Autodesk Fusion 360 part; units mm, degrees
(part 39 of 40)
  line L11251 (159.0031, 181.5729) -> (158.8856, 181.6744) construction
  line L11252 (158.8856, 181.6744) -> (158.7686, 181.7767) construction
  line L11253 (158.7686, 181.7767) -> (158.6523, 181.88) construction
  line L11254 (158.6523, 181.88) -> (158.5369, 181.9844) construction
  line L11255 (158.5369, 181.9844) -> (158.4226, 182.0903) construction
  line L11256 (158.4226, 182.0903) -> (158.3096, 182.1981) construction
  line L11257 (158.3096, 182.1981) -> (158.198, 182.3077) construction
  line L11258 (158.198, 182.3077) -> (158.0876, 182.419) construction
  line L11259 (158.0876, 182.419) -> (157.9783, 182.5316) construction
  line L11260 (157.9783, 182.5316) -> (157.8698, 182.6455) construction
  line L11261 (157.8698, 182.6455) -> (157.7622, 182.7603) construction
  line L11262 (157.7622, 182.7603) -> (157.6553, 182.876) construction
  line L11263 (157.6553, 182.876) -> (157.5492, 182.9927) construction
  line L11264 (157.5492, 182.9927) -> (157.4439, 183.1105) construction
  line L11265 (157.4439, 183.1105) -> (157.3394, 183.2292) construction
  line L11266 (157.3394, 183.2292) -> (157.2359, 183.3491) construction
  line L11267 (157.2359, 183.3491) -> (157.1332, 183.47) construction
  line L11268 (157.1332, 183.47) -> (157.0313, 183.5919) construction
  line L11269 (157.0313, 183.5919) -> (156.9303, 183.7148) construction
  line L11270 (156.9303, 183.7148) -> (156.83, 183.8386) construction
  line L11271 (156.83, 183.8386) -> (156.7305, 183.9633) construction
  line L11272 (156.7305, 183.9633) -> (156.6317, 184.0888) construction
  line L11273 (156.6317, 184.0888) -> (156.5336, 184.2151) construction
  line L11274 (156.5336, 184.2151) -> (156.4363, 184.3423) construction
  line L11275 (156.4363, 184.3423) -> (156.3397, 184.4703) construction
  line L11276 (156.3397, 184.4703) -> (156.2439, 184.5991) construction
  line L11277 (156.2439, 184.5991) -> (156.1488, 184.7288) construction
  line L11278 (156.1488, 184.7288) -> (156.0544, 184.8592) construction
  line L11279 (156.0544, 184.8592) -> (155.9608, 184.9905) construction
  line L11280 (155.9608, 184.9905) -> (155.8678, 185.1224) construction
  line L11281 (155.8678, 185.1224) -> (155.7756, 185.2552) construction
  line L11282 (155.7756, 185.2552) -> (155.684, 185.3886) construction
  line L11283 (155.684, 185.3886) -> (155.5932, 185.5228) construction
  line L11284 (155.5932, 185.5228) -> (155.503, 185.6577) construction
  line L11285 (155.503, 185.6577) -> (155.4135, 185.7933) construction
  line L11286 (155.4135, 185.7933) -> (155.3247, 185.9295) construction
  line L11287 (155.3247, 185.9295) -> (155.2365, 186.0665) construction
  line L11288 (155.2365, 186.0665) -> (155.1491, 186.2042) construction
  line L11289 (155.1491, 186.2042) -> (155.0623, 186.3425) construction
  line L11290 (155.0623, 186.3425) -> (154.9762, 186.4815) construction
  line L11291 (154.9762, 186.4815) -> (154.8907, 186.6211) construction
  line L11292 (154.8907, 186.6211) -> (154.8059, 186.7614) construction
  line L11293 (154.8059, 186.7614) -> (154.7218, 186.9023) construction
  line L11294 (154.7218, 186.9023) -> (154.6383, 187.0438) construction
  line L11295 (154.6383, 187.0438) -> (154.5555, 187.186) construction
  line L11296 (154.5555, 187.186) -> (154.4733, 187.3288) construction
  line L11297 (154.4733, 187.3288) -> (154.3917, 187.4721) construction
  line L11298 (154.3917, 187.4721) -> (154.3108, 187.6161) construction
  line L11299 (154.3108, 187.6161) -> (154.2306, 187.7607) construction
  line L11300 (154.2306, 187.7607) -> (154.151, 187.9058) construction
  line L11301 (154.151, 187.9058) -> (154.072, 188.0515) construction
  line L11302 (154.072, 188.0515) -> (153.9937, 188.1978) construction
  line L11303 (153.9937, 188.1978) -> (153.916, 188.3447) construction
  line L11304 (153.916, 188.3447) -> (153.8389, 188.4921) construction
  line L11305 (153.8389, 188.4921) -> (153.7625, 188.6401) construction
  line L11306 (153.7625, 188.6401) -> (153.6867, 188.7886) construction
  line L11307 (153.6867, 188.7886) -> (153.6115, 188.9377) construction
  line L11308 (153.6115, 188.9377) -> (153.537, 189.0873) construction
  line L11309 (153.537, 189.0873) -> (153.463, 189.2374) construction
  line L11310 (153.463, 189.2374) -> (153.3897, 189.3881) construction
  line L11311 (153.3897, 189.3881) -> (153.3171, 189.5393) construction
  line L11312 (153.3171, 189.5393) -> (153.245, 189.6909) construction
  line L11313 (153.245, 189.6909) -> (153.1736, 189.8431) construction
  line L11314 (153.1736, 189.8431) -> (153.1169, 189.9653) construction
  line L11315 (153.1169, 189.9653) -> (153.0747, 190.0572) construction
  line L11316 (153.0747, 190.0572) -> (153.0467, 190.1185) construction
  line L11317 (153.0467, 190.1185) -> (153.0327, 190.1492) construction
  line L11318 (256.7226, 110.7517) -> (257.9473, 109.6737)
  line L11319 (154.1697, 136.995) -> (152.5778, 136.6378)
  line L11320 (154.1697, 163.005) -> (152.5778, 163.3622)
  line L11321 (217.6748, 90.8558) -> (217.8271, 89.2315)
  line L11322 (152.9878, 144.4572) -> (151.3635, 144.3049)
  line L11323 (225.137, 92.0377) -> (225.4942, 90.4458)
  line L11324 (266.6686, 173.5481) -> (268.1665, 174.1948)
  line L11325 (263.2386, 119.7202) -> (264.6423, 118.8885)
  line L11326 (270.0943, 136.995) -> (271.6862, 136.6378)
  line L11327 (242.4118, 201.1066) -> (243.2435, 202.5103)
  line L11328 (161.0254, 180.2798) -> (159.6217, 181.1115)
  line L11329 (154.1697, 136.995) -> (152.5778, 136.6378)
  arc A302 (172.7536, 191.8132) -> (172.8837, 194.5906) centre (171.3824, 193.2692) ccw
  arc A303 (199.127, 207.9623) -> (201.4504, 206.435) centre (201.0785, 208.4001) ccw
  arc A304 (204.8514, 206.9737) -> (206.5892, 209.1442) centre (204.5979, 208.9575) ccw
  arc A305 (239.7302, 200.3721) -> (242.4118, 201.1066) centre (240.6912, 202.1261) ccw
  arc A306 (266.6686, 126.4519) -> (264.0674, 125.4699) centre (265.8758, 124.6158) ccw
  arc A307 (256.7226, 110.7517) -> (253.9452, 110.6216) centre (255.4012, 109.2504) ccw
  spline S151 degree 5 poles (198.7698, 90.4458) (198.763, 90.4157) (198.7487, 90.3556) (198.7249, 90.2662) (198.6885, 90.1483) (198.6369, 90.0027) (198.5809, 89.8584) (198.5221, 89.7148) (198.4619, 89.5717) (198.4007, 89.4289) (198.3385, 89.2864) (198.2749, 89.1443) (198.2094, 89.0029) (198.1418, 88.8621) (198.072, 88.7221) (198.0004, 88.5827) (197.927, 88.4439) (197.8523, 88.3056) (197.7763, 88.1678) (197.6993, 88.0303) (197.6211, 87.8933) (197.5416, 87.7568) (197.4609, 87.6208) (197.379, 87.4852) (197.2957, 87.3502) (197.2112, 87.2157) (197.1256, 87.0816) (197.0388, 86.948) (196.951, 86.8148) (196.8622, 86.682) (196.7723, 86.5497) (196.6814, 86.4179) (196.5895, 86.2865) (196.4966, 86.1555) (196.4027, 86.025) (196.3078, 85.895) (196.212, 85.7654) (196.1152, 85.6362) (196.0174, 85.5074) (195.9188, 85.3791) (195.8193, 85.2512) (195.7189, 85.1238) (195.6176, 84.9968) (195.5154, 84.8702) (195.4124, 84.744) (195.3085, 84.6183) (195.2037, 84.493) (195.0982, 84.3682) (194.9918, 84.2438) (194.8846, 84.1198) (194.7765, 83.9962) (194.6677, 83.8731) (194.5581, 83.7503) (194.4478, 83.6281) (194.3366, 83.5062) (194.2247, 83.3848) (194.112, 83.2638) (193.9985, 83.1432) (193.8843, 83.0231) (193.7694, 82.9034) (193.6538, 82.7841) (193.5374, 82.6653) (193.4202, 82.5469) (193.3024, 82.4289) (193.1839, 82.3113) (193.0646, 82.1942) (192.9447, 82.0775) (192.8241, 81.9612) (192.7027, 81.8454) (192.5808, 81.73) (192.4581, 81.615) (192.3594, 81.5233) (192.2851, 81.4548) (192.2354, 81.4092) (192.2105, 81.3864) knots 0 0 0 0 0 0 0.01428571 0.02857143 0.04285714 0.05714286 0.07142857 0.08571429 0.1 0.11428571 0.12857143 0.14285714 0.15714286 0.17142857 0.18571429 0.2 0.21428571 0.22857143 0.24285714 0.25714286 0.27142857 0.28571429 0.3 0.31428571 0.32857143 0.34285714 0.35714286 0.37142857 0.38571429 0.4 0.41428571 0.42857143 0.44285714 0.45714286 0.47142857 0.48571429 0.5 0.51428571 0.52857143 0.54285714 0.55714286 0.57142857 0.58571429 0.6 0.61428571 0.62857143 0.64285714 0.65714286 0.67142857 0.68571429 0.7 0.71428571 0.72857143 0.74285714 0.75714286 0.77142857 0.78571429 0.8 0.81428571 0.82857143 0.84285714 0.85714286 0.87142857 0.88571429 0.9 0.91428571 0.92857143 0.94285714 0.95714286 0.97142857 0.98571429 1 1 1 1 1 1
  line L11330 (198.7698, 90.4458) -> (198.763, 90.4157) construction
  line L11331 (198.763, 90.4157) -> (198.7487, 90.3556) construction
  line L11332 (198.7487, 90.3556) -> (198.7249, 90.2662) construction
  line L11333 (198.7249, 90.2662) -> (198.6885, 90.1483) construction
  line L11334 (198.6885, 90.1483) -> (198.6369, 90.0027) construction
  line L11335 (198.6369, 90.0027) -> (198.5809, 89.8584) construction
  line L11336 (198.5809, 89.8584) -> (198.5221, 89.7148) construction
  line L11337 (198.5221, 89.7148) -> (198.4619, 89.5717) construction
  line L11338 (198.4619, 89.5717) -> (198.4007, 89.4289) construction
  line L11339 (198.4007, 89.4289) -> (198.3385, 89.2864) construction
  line L11340 (198.3385, 89.2864) -> (198.2749, 89.1443) construction
  line L11341 (198.2749, 89.1443) -> (198.2094, 89.0029) construction
  line L11342 (198.2094, 89.0029) -> (198.1418, 88.8621) construction
  line L11343 (198.1418, 88.8621) -> (198.072, 88.7221) construction
  line L11344 (198.072, 88.7221) -> (198.0004, 88.5827) construction
  line L11345 (198.0004, 88.5827) -> (197.927, 88.4439) construction
  line L11346 (197.927, 88.4439) -> (197.8523, 88.3056) construction
  line L11347 (197.8523, 88.3056) -> (197.7763, 88.1678) construction
  line L11348 (197.7763, 88.1678) -> (197.6993, 88.0303) construction
  line L11349 (197.6993, 88.0303) -> (197.6211, 87.8933) construction
  line L11350 (197.6211, 87.8933) -> (197.5416, 87.7568) construction
  line L11351 (197.5416, 87.7568) -> (197.4609, 87.6208) construction
  line L11352 (197.4609, 87.6208) -> (197.379, 87.4852) construction
  line L11353 (197.379, 87.4852) -> (197.2957, 87.3502) construction
  line L11354 (197.2957, 87.3502) -> (197.2112, 87.2157) construction
  line L11355 (197.2112, 87.2157) -> (197.1256, 87.0816) construction
  line L11356 (197.1256, 87.0816) -> (197.0388, 86.948) construction
  line L11357 (197.0388, 86.948) -> (196.951, 86.8148) construction
  line L11358 (196.951, 86.8148) -> (196.8622, 86.682) construction
  line L11359 (196.8622, 86.682) -> (196.7723, 86.5497) construction
  line L11360 (196.7723, 86.5497) -> (196.6814, 86.4179) construction
  line L11361 (196.6814, 86.4179) -> (196.5895, 86.2865) construction
  line L11362 (196.5895, 86.2865) -> (196.4966, 86.1555) construction
  line L11363 (196.4966, 86.1555) -> (196.4027, 86.025) construction
  line L11364 (196.4027, 86.025) -> (196.3078, 85.895) construction
  line L11365 (196.3078, 85.895) -> (196.212, 85.7654) construction
  line L11366 (196.212, 85.7654) -> (196.1152, 85.6362) construction
  line L11367 (196.1152, 85.6362) -> (196.0174, 85.5074) construction
  line L11368 (196.0174, 85.5074) -> (195.9188, 85.3791) construction
  line L11369 (195.9188, 85.3791) -> (195.8193, 85.2512) construction
  line L11370 (195.8193, 85.2512) -> (195.7189, 85.1238) construction
  line L11371 (195.7189, 85.1238) -> (195.6176, 84.9968) construction
  line L11372 (195.6176, 84.9968) -> (195.5154, 84.8702) construction
  line L11373 (195.5154, 84.8702) -> (195.4124, 84.744) construction
  line L11374 (195.4124, 84.744) -> (195.3085, 84.6183) construction
  line L11375 (195.3085, 84.6183) -> (195.2037, 84.493) construction
  line L11376 (195.2037, 84.493) -> (195.0982, 84.3682) construction
  line L11377 (195.0982, 84.3682) -> (194.9918, 84.2438) construction
  line L11378 (194.9918, 84.2438) -> (194.8846, 84.1198) construction
  line L11379 (194.8846, 84.1198) -> (194.7765, 83.9962) construction
  line L11380 (194.7765, 83.9962) -> (194.6677, 83.8731) construction
  line L11381 (194.6677, 83.8731) -> (194.5581, 83.7503) construction
  line L11382 (194.5581, 83.7503) -> (194.4478, 83.6281) construction
  line L11383 (194.4478, 83.6281) -> (194.3366, 83.5062) construction
  line L11384 (194.3366, 83.5062) -> (194.2247, 83.3848) construction
  line L11385 (194.2247, 83.3848) -> (194.112, 83.2638) construction
  line L11386 (194.112, 83.2638) -> (193.9985, 83.1432) construction
  line L11387 (193.9985, 83.1432) -> (193.8843, 83.0231) construction
  line L11388 (193.8843, 83.0231) -> (193.7694, 82.9034) construction
  line L11389 (193.7694, 82.9034) -> (193.6538, 82.7841) construction
  line L11390 (193.6538, 82.7841) -> (193.5374, 82.6653) construction
  line L11391 (193.5374, 82.6653) -> (193.4202, 82.5469) construction
  line L11392 (193.4202, 82.5469) -> (193.3024, 82.4289) construction
  line L11393 (193.3024, 82.4289) -> (193.1839, 82.3113) construction
  line L11394 (193.1839, 82.3113) -> (193.0646, 82.1942) construction
  line L11395 (193.0646, 82.1942) -> (192.9447, 82.0775) construction
  line L11396 (192.9447, 82.0775) -> (192.8241, 81.9612) construction
  line L11397 (192.8241, 81.9612) -> (192.7027, 81.8454) construction
  line L11398 (192.7027, 81.8454) -> (192.5808, 81.73) construction
  line L11399 (192.5808, 81.73) -> (192.4581, 81.615) construction
  line L11400 (192.4581, 81.615) -> (192.3594, 81.5233) construction
  line L11401 (192.3594, 81.5233) -> (192.2851, 81.4548) construction
  line L11402 (192.2851, 81.4548) -> (192.2354, 81.4092) construction
  line L11403 (192.2354, 81.4092) -> (192.2105, 81.3864) construction
  spline S152 degree 5 poles (159.6217, 118.8885) (159.5952, 118.8728) (159.5425, 118.8406) (159.4648, 118.7903) (159.3639, 118.7193) (159.2414, 118.6252) (159.1214, 118.5273) (159.0031, 118.4271) (158.8856, 118.3256) (158.7686, 118.2233) (158.6523, 118.12) (158.5369, 118.0156) (158.4226, 117.9097) (158.3096, 117.8019) (158.198, 117.6923) (158.0876, 117.581) (157.9783, 117.4684) (157.8698, 117.3545) (157.7622, 117.2397) (157.6553, 117.124) (157.5492, 117.0073) (157.4439, 116.8895) (157.3394, 116.7708) (157.2359, 116.6509) (157.1332, 116.53) (157.0313, 116.4081) (156.9303, 116.2852) (156.83, 116.1614) (156.7305, 116.0367) (156.6317, 115.9112) (156.5336, 115.7849) (156.4363, 115.6577) (156.3397, 115.5297) (156.2439, 115.4009) (156.1488, 115.2712) (156.0544, 115.1408) (155.9608, 115.0095) (155.8678, 114.8776) (155.7756, 114.7448) (155.684, 114.6114) (155.5932, 114.4772) (155.503, 114.3423) (155.4135, 114.2067) (155.3247, 114.0705) (155.2365, 113.9335) (155.1491, 113.7958) (155.0623, 113.6575) (154.9762, 113.5185) (154.8907, 113.3789) (154.8059, 113.2386) (154.7218, 113.0977) (154.6383, 112.9562) (154.5555, 112.814) (154.4733, 112.6712) (154.3917, 112.5279) (154.3108, 112.3839) (154.2306, 112.2393) (154.151, 112.0942) (154.072, 111.9485) (153.9937, 111.8022) (153.916, 111.6553) (153.8389, 111.5079) (153.7625, 111.3599) (153.6867, 111.2114) (153.6115, 111.0623) (153.537, 110.9127) (153.463, 110.7626) (153.3897, 110.6119) (153.3171, 110.4607) (153.245, 110.3091) (153.1736, 110.1569) (153.1169, 110.0347) (153.0747, 109.9428) (153.0467, 109.8815) (153.0327, 109.8508) knots 0 0 0 0 0 0 0.01428571 0.02857143 0.04285714 0.05714286 0.07142857 0.08571429 0.1 0.11428571 0.12857143 0.14285714 0.15714286 0.17142857 0.18571429 0.2 0.21428571 0.22857143 0.24285714 0.25714286 0.27142857 0.28571429 0.3 0.31428571 0.32857143 0.34285714 0.35714286 0.37142857 0.38571429 0.4 0.41428571 0.42857143 0.44285714 0.45714286 0.47142857 0.48571429 0.5 0.51428571 0.52857143 0.54285714 0.55714286 0.57142857 0.58571429 0.6 0.61428571 0.62857143 0.64285714 0.65714286 0.67142857 0.68571429 0.7 0.71428571 0.72857143 0.74285714 0.75714286 0.77142857 0.78571429 0.8 0.81428571 0.82857143 0.84285714 0.85714286 0.87142857 0.88571429 0.9 0.91428571 0.92857143 0.94285714 0.95714286 0.97142857 0.98571429 1 1 1 1 1 1
  line L11404 (159.6217, 118.8885) -> (159.5952, 118.8728) construction
  line L11405 (159.5952, 118.8728) -> (159.5425, 118.8406) construction
  line L11406 (159.5425, 118.8406) -> (159.4648, 118.7903) construction
  line L11407 (159.4648, 118.7903) -> (159.3639, 118.7193) construction
  line L11408 (159.3639, 118.7193) -> (159.2414, 118.6252) construction
  line L11409 (159.2414, 118.6252) -> (159.1214, 118.5273) construction
  line L11410 (159.1214, 118.5273) -> (159.0031, 118.4271) construction
  line L11411 (159.0031, 118.4271) -> (158.8856, 118.3256) construction
  line L11412 (158.8856, 118.3256) -> (158.7686, 118.2233) construction
  line L11413 (158.7686, 118.2233) -> (158.6523, 118.12) construction
  line L11414 (158.6523, 118.12) -> (158.5369, 118.0156) construction
  line L11415 (158.5369, 118.0156) -> (158.4226, 117.9097) construction
  line L11416 (158.4226, 117.9097) -> (158.3096, 117.8019) construction
  line L11417 (158.3096, 117.8019) -> (158.198, 117.6923) construction
  line L11418 (158.198, 117.6923) -> (158.0876, 117.581) construction
  line L11419 (158.0876, 117.581) -> (157.9783, 117.4684) construction
  line L11420 (157.9783, 117.4684) -> (157.8698, 117.3545) construction
  line L11421 (157.8698, 117.3545) -> (157.7622, 117.2397) construction
  line L11422 (157.7622, 117.2397) -> (157.6553, 117.124) construction
  line L11423 (157.6553, 117.124) -> (157.5492, 117.0073) construction
  line L11424 (157.5492, 117.0073) -> (157.4439, 116.8895) construction
  line L11425 (157.4439, 116.8895) -> (157.3394, 116.7708) construction
  line L11426 (157.3394, 116.7708) -> (157.2359, 116.6509) construction
  line L11427 (157.2359, 116.6509) -> (157.1332, 116.53) construction
  line L11428 (157.1332, 116.53) -> (157.0313, 116.4081) construction
  line L11429 (157.0313, 116.4081) -> (156.9303, 116.2852) construction
  line L11430 (156.9303, 116.2852) -> (156.83, 116.1614) construction
  line L11431 (156.83, 116.1614) -> (156.7305, 116.0367) construction
  line L11432 (156.7305, 116.0367) -> (156.6317, 115.9112) construction
  line L11433 (156.6317, 115.9112) -> (156.5336, 115.7849) construction
  line L11434 (156.5336, 115.7849) -> (156.4363, 115.6577) construction
  line L11435 (156.4363, 115.6577) -> (156.3397, 115.5297) construction
  line L11436 (156.3397, 115.5297) -> (156.2439, 115.4009) construction
  line L11437 (156.2439, 115.4009) -> (156.1488, 115.2712) construction
  line L11438 (156.1488, 115.2712) -> (156.0544, 115.1408) construction
  line L11439 (156.0544, 115.1408) -> (155.9608, 115.0095) construction
  line L11440 (155.9608, 115.0095) -> (155.8678, 114.8776) construction
  line L11441 (155.8678, 114.8776) -> (155.7756, 114.7448) construction
  line L11442 (155.7756, 114.7448) -> (155.684, 114.6114) construction
  line L11443 (155.684, 114.6114) -> (155.5932, 114.4772) construction
  line L11444 (155.5932, 114.4772) -> (155.503, 114.3423) construction
  line L11445 (155.503, 114.3423) -> (155.4135, 114.2067) construction
  line L11446 (155.4135, 114.2067) -> (155.3247, 114.0705) construction
  line L11447 (155.3247, 114.0705) -> (155.2365, 113.9335) construction
  line L11448 (155.2365, 113.9335) -> (155.1491, 113.7958) construction
  line L11449 (155.1491, 113.7958) -> (155.0623, 113.6575) construction
  line L11450 (155.0623, 113.6575) -> (154.9762, 113.5185) construction
  line L11451 (154.9762, 113.5185) -> (154.8907, 113.3789) construction
  line L11452 (154.8907, 113.3789) -> (154.8059, 113.2386) construction
  line L11453 (154.8059, 113.2386) -> (154.7218, 113.0977) construction
  line L11454 (154.7218, 113.0977) -> (154.6383, 112.9562) construction
  line L11455 (154.6383, 112.9562) -> (154.5555, 112.814) construction
  line L11456 (154.5555, 112.814) -> (154.4733, 112.6712) construction
  line L11457 (154.4733, 112.6712) -> (154.3917, 112.5279) construction
  line L11458 (154.3917, 112.5279) -> (154.3108, 112.3839) construction
  line L11459 (154.3108, 112.3839) -> (154.2306, 112.2393) construction
  line L11460 (154.2306, 112.2393) -> (154.151, 112.0942) construction
  line L11461 (154.151, 112.0942) -> (154.072, 111.9485) construction
  line L11462 (154.072, 111.9485) -> (153.9937, 111.8022) construction
  line L11463 (153.9937, 111.8022) -> (153.916, 111.6553) construction
  line L11464 (153.916, 111.6553) -> (153.8389, 111.5079) construction
  line L11465 (153.8389, 111.5079) -> (153.7625, 111.3599) construction
  line L11466 (153.7625, 111.3599) -> (153.6867, 111.2114) construction
  line L11467 (153.6867, 111.2114) -> (153.6115, 111.0623) construction
  line L11468 (153.6115, 111.0623) -> (153.537, 110.9127) construction
  line L11469 (153.537, 110.9127) -> (153.463, 110.7626) construction
  line L11470 (153.463, 110.7626) -> (153.3897, 110.6119) construction
  line L11471 (153.3897, 110.6119) -> (153.3171, 110.4607) construction
  line L11472 (153.3171, 110.4607) -> (153.245, 110.3091) construction
  line L11473 (153.245, 110.3091) -> (153.1736, 110.1569) construction
  line L11474 (153.1736, 110.1569) -> (153.1169, 110.0347) construction
  line L11475 (153.1169, 110.0347) -> (153.0747, 109.9428) construction
  line L11476 (153.0747, 109.9428) -> (153.0467, 109.8815) construction
  line L11477 (153.0467, 109.8815) -> (153.0327, 109.8508) construction
  arc A308 (144.9129, 174.2132) -> (143.5184, 169.9215) centre (212.132, 150) ccw
  spline S153 degree 5 poles (171.8057, 104.1847) (171.7853, 104.1615) (171.7452, 104.1146) (171.6869, 104.0427) (171.6128, 103.944) (171.5254, 103.8167) (171.4416, 103.6865) (171.36, 103.5546) (171.2796, 103.4218) (171.2, 103.2883) (171.1213, 103.1542) (171.0437, 103.0193) (170.9678, 102.8832) (170.8937, 102.7457) (170.8214, 102.607) (170.7507, 102.4671) (170.6816, 102.3262) (170.6136, 102.1844) (170.5467, 102.0419) (170.4808, 101.8988) (170.416, 101.755) (170.3522, 101.6105) (170.2896, 101.4653) (170.2281, 101.3193) (170.1678, 101.1726) (170.1086, 101.0251) (170.0505, 100.877) (169.9934, 100.7283) (169.9373, 100.579) (169.8821, 100.4291) (169.8279, 100.2786) (169.7746, 100.1276) (169.7223, 99.976) (169.671, 99.8239) (169.6206, 99.6712) (169.5712, 99.518) (169.5226, 99.3642) (169.475, 99.21) (169.4283, 99.0553) (169.3825, 98.9001) (169.3375, 98.7444) (169.2934, 98.5882) (169.2502, 98.4316) (169.2079, 98.2745) (169.1664, 98.117) (169.1257, 97.9591) (169.0859, 97.8007) (169.047, 97.6419) (169.0089, 97.4827) (168.9716, 97.3231) (168.9351, 97.1631) (168.8994, 97.0027) (168.8646, 96.8419) (168.8305, 96.6807) (168.7973, 96.5191) (168.7648, 96.3572) (168.7332, 96.1949) (168.7023, 96.0323) (168.6723, 95.8693) (168.643, 95.706) (168.6145, 95.5423) (168.5867, 95.3783) (168.5597, 95.2139) (168.5336, 95.0492) (168.5081, 94.8842) (168.4834, 94.7189) (168.4595, 94.5533) (168.4364, 94.3874) (168.414, 94.2211) (168.3923, 94.0546) (168.3714, 93.8878) (168.3553, 93.7541) (168.3435, 93.6537) (168.3358, 93.5867) (168.332, 93.5531) knots 0 0 0 0 0 0 0.01428571 0.02857143 0.04285714 0.05714286 0.07142857 0.08571429 0.1 0.11428571 0.12857143 0.14285714 0.15714286 0.17142857 0.18571429 0.2 0.21428571 0.22857143 0.24285714 0.25714286 0.27142857 0.28571429 0.3 0.31428571 0.32857143 0.34285714 0.35714286 0.37142857 0.38571429 0.4 0.41428571 0.42857143 0.44285714 0.45714286 0.47142857 0.48571429 0.5 0.51428571 0.52857143 0.54285714 0.55714286 0.57142857 0.58571429 0.6 0.61428571 0.62857143 0.64285714 0.65714286 0.67142857 0.68571429 0.7 0.71428571 0.72857143 0.74285714 0.75714286 0.77142857 0.78571429 0.8 0.81428571 0.82857143 0.84285714 0.85714286 0.87142857 0.88571429 0.9 0.91428571 0.92857143 0.94285714 0.95714286 0.97142857 0.98571429 1 1 1 1 1 1
  line L11478 (171.8057, 104.1847) -> (171.7853, 104.1615) construction
  line L11479 (171.7853, 104.1615) -> (171.7452, 104.1146) construction
  line L11480 (171.7452, 104.1146) -> (171.6869, 104.0427) construction
  line L11481 (171.6869, 104.0427) -> (171.6128, 103.944) construction
  line L11482 (171.6128, 103.944) -> (171.5254, 103.8167) construction
  line L11483 (171.5254, 103.8167) -> (171.4416, 103.6865) construction
  line L11484 (171.4416, 103.6865) -> (171.36, 103.5546) construction
  line L11485 (171.36, 103.5546) -> (171.2796, 103.4218) construction
  line L11486 (171.2796, 103.4218) -> (171.2, 103.2883) construction
  line L11487 (171.2, 103.2883) -> (171.1213, 103.1542) construction
  line L11488 (171.1213, 103.1542) -> (171.0437, 103.0193) construction
  line L11489 (171.0437, 103.0193) -> (170.9678, 102.8832) construction
  line L11490 (170.9678, 102.8832) -> (170.8937, 102.7457) construction
  line L11491 (170.8937, 102.7457) -> (170.8214, 102.607) construction
  line L11492 (170.8214, 102.607) -> (170.7507, 102.4671) construction
  line L11493 (170.7507, 102.4671) -> (170.6816, 102.3262) construction
  line L11494 (170.6816, 102.3262) -> (170.6136, 102.1844) construction
  line L11495 (170.6136, 102.1844) -> (170.5467, 102.0419) construction
  line L11496 (170.5467, 102.0419) -> (170.4808, 101.8988) construction
  line L11497 (170.4808, 101.8988) -> (170.416, 101.755) construction
  line L11498 (170.416, 101.755) -> (170.3522, 101.6105) construction
  line L11499 (170.3522, 101.6105) -> (170.2896, 101.4653) construction
  line L11500 (170.2896, 101.4653) -> (170.2281, 101.3193) construction
  line L11501 (170.2281, 101.3193) -> (170.1678, 101.1726) construction
  line L11502 (170.1678, 101.1726) -> (170.1086, 101.0251) construction
  line L11503 (170.1086, 101.0251) -> (170.0505, 100.877) construction
  line L11504 (170.0505, 100.877) -> (169.9934, 100.7283) construction
  line L11505 (169.9934, 100.7283) -> (169.9373, 100.579) construction
  line L11506 (169.9373, 100.579) -> (169.8821, 100.4291) construction
  line L11507 (169.8821, 100.4291) -> (169.8279, 100.2786) construction
  line L11508 (169.8279, 100.2786) -> (169.7746, 100.1276) construction
  line L11509 (169.7746, 100.1276) -> (169.7223, 99.976) construction
  line L11510 (169.7223, 99.976) -> (169.671, 99.8239) construction
  line L11511 (169.671, 99.8239) -> (169.6206, 99.6712) construction
  line L11512 (169.6206, 99.6712) -> (169.5712, 99.518) construction
  line L11513 (169.5712, 99.518) -> (169.5226, 99.3642) construction
  line L11514 (169.5226, 99.3642) -> (169.475, 99.21) construction
  line L11515 (169.475, 99.21) -> (169.4283, 99.0553) construction
  line L11516 (169.4283, 99.0553) -> (169.3825, 98.9001) construction
  line L11517 (169.3825, 98.9001) -> (169.3375, 98.7444) construction
  line L11518 (169.3375, 98.7444) -> (169.2934, 98.5882) construction
  line L11519 (169.2934, 98.5882) -> (169.2502, 98.4316) construction
  line L11520 (169.2502, 98.4316) -> (169.2079, 98.2745) construction
  line L11521 (169.2079, 98.2745) -> (169.1664, 98.117) construction
  line L11522 (169.1664, 98.117) -> (169.1257, 97.9591) construction
  line L11523 (169.1257, 97.9591) -> (169.0859, 97.8007) construction
  line L11524 (169.0859, 97.8007) -> (169.047, 97.6419) construction
  line L11525 (169.047, 97.6419) -> (169.0089, 97.4827) construction
  line L11526 (169.0089, 97.4827) -> (168.9716, 97.3231) construction
  line L11527 (168.9716, 97.3231) -> (168.9351, 97.1631) construction
  line L11528 (168.9351, 97.1631) -> (168.8994, 97.0027) construction
  line L11529 (168.8994, 97.0027) -> (168.8646, 96.8419) construction
  line L11530 (168.8646, 96.8419) -> (168.8305, 96.6807) construction
  line L11531 (168.8305, 96.6807) -> (168.7973, 96.5191) construction
  line L11532 (168.7973, 96.5191) -> (168.7648, 96.3572) construction
  line L11533 (168.7648, 96.3572) -> (168.7332, 96.1949) construction
  line L11534 (168.7332, 96.1949) -> (168.7023, 96.0323) construction
  line L11535 (168.7023, 96.0323) -> (168.6723, 95.8693) construction
  line L11536 (168.6723, 95.8693) -> (168.643, 95.706) construction
  line L11537 (168.643, 95.706) -> (168.6145, 95.5423) construction
  line L11538 (168.6145, 95.5423) -> (168.5867, 95.3783) construction
  line L11539 (168.5867, 95.3783) -> (168.5597, 95.2139) construction
  line L11540 (168.5597, 95.2139) -> (168.5336, 95.0492) construction
  line L11541 (168.5336, 95.0492) -> (168.5081, 94.8842) construction
  line L11542 (168.5081, 94.8842) -> (168.4834, 94.7189) construction
  line L11543 (168.4834, 94.7189) -> (168.4595, 94.5533) construction
  line L11544 (168.4595, 94.5533) -> (168.4364, 94.3874) construction
  line L11545 (168.4364, 94.3874) -> (168.414, 94.2211) construction
  line L11546 (168.414, 94.2211) -> (168.3923, 94.0546) construction
  line L11547 (168.3923, 94.0546) -> (168.3714, 93.8878) construction
  line L11548 (168.3714, 93.8878) -> (168.3553, 93.7541) construction
  line L11549 (168.3553, 93.7541) -> (168.3435, 93.6537) construction
  line L11550 (168.3435, 93.6537) -> (168.3358, 93.5867) construction
  line L11551 (168.3358, 93.5867) -> (168.332, 93.5531) construction
  spline S154 degree 5 poles (171.8057, 195.8153) (171.7853, 195.8385) (171.7452, 195.8854) (171.6869, 195.9573) (171.6128, 196.056) (171.5254, 196.1833) (171.4416, 196.3135) (171.36, 196.4454) (171.2796, 196.5782) (171.2, 196.7117) (171.1213, 196.8458) (171.0437, 196.9807) (170.9678, 197.1168) (170.8937, 197.2543) (170.8214, 197.393) (170.7507, 197.5329) (170.6816, 197.6738) (170.6136, 197.8156) (170.5467, 197.9581) (170.4808, 198.1012) (170.416, 198.245) (170.3522, 198.3895) (170.2896, 198.5347) (170.2281, 198.6807) (170.1678, 198.8274) (170.1086, 198.9749) (170.0505, 199.123) (169.9934, 199.2717) (169.9373, 199.421) (169.8821, 199.5709) (169.8279, 199.7214) (169.7746, 199.8724) (169.7223, 200.024) (169.671, 200.1761) (169.6206, 200.3288) (169.5712, 200.482) (169.5226, 200.6358) (169.475, 200.79) (169.4283, 200.9447) (169.3825, 201.0999) (169.3375, 201.2556) (169.2934, 201.4118) (169.2502, 201.5684) (169.2079, 201.7255) (169.1664, 201.883) (169.1257, 202.0409) (169.0859, 202.1993) (169.047, 202.3581) (169.0089, 202.5173) (168.9716, 202.6769) (168.9351, 202.8369) (168.8994, 202.9973) (168.8646, 203.1581) (168.8305, 203.3193) (168.7973, 203.4809) (168.7648, 203.6428) (168.7332, 203.8051) (168.7023, 203.9677) (168.6723, 204.1307) (168.643, 204.294) (168.6145, 204.4577) (168.5867, 204.6217) (168.5597, 204.7861) (168.5336, 204.9508) (168.5081, 205.1158) (168.4834, 205.2811) (168.4595, 205.4467) (168.4364, 205.6126) (168.414, 205.7789) (168.3923, 205.9454) (168.3714, 206.1122) (168.3553, 206.2459) (168.3435, 206.3463) (168.3358, 206.4133) (168.332, 206.4469) knots 0 0 0 0 0 0 0.01428571 0.02857143 0.04285714 0.05714286 0.07142857 0.08571429 0.1 0.11428571 0.12857143 0.14285714 0.15714286 0.17142857 0.18571429 0.2 0.21428571 0.22857143 0.24285714 0.25714286 0.27142857 0.28571429 0.3 0.31428571 0.32857143 0.34285714 0.35714286 0.37142857 0.38571429 0.4 0.41428571 0.42857143 0.44285714 0.45714286 0.47142857 0.48571429 0.5 0.51428571 0.52857143 0.54285714 0.55714286 0.57142857 0.58571429 0.6 0.61428571 0.62857143 0.64285714 0.65714286 0.67142857 0.68571429 0.7 0.71428571 0.72857143 0.74285714 0.75714286 0.77142857 0.78571429 0.8 0.81428571 0.82857143 0.84285714 0.85714286 0.87142857 0.88571429 0.9 0.91428571 0.92857143 0.94285714 0.95714286 0.97142857 0.98571429 1 1 1 1 1 1
  line L11552 (171.8057, 195.8153) -> (171.7853, 195.8385) construction
  line L11553 (171.7853, 195.8385) -> (171.7452, 195.8854) construction
  line L11554 (171.7452, 195.8854) -> (171.6869, 195.9573) construction
  line L11555 (171.6869, 195.9573) -> (171.6128, 196.056) construction
  line L11556 (171.6128, 196.056) -> (171.5254, 196.1833) construction
  line L11557 (171.5254, 196.1833) -> (171.4416, 196.3135) construction
  line L11558 (171.4416, 196.3135) -> (171.36, 196.4454) construction
  line L11559 (171.36, 196.4454) -> (171.2796, 196.5782) construction
  line L11560 (171.2796, 196.5782) -> (171.2, 196.7117) construction
  line L11561 (171.2, 196.7117) -> (171.1213, 196.8458) construction
  line L11562 (171.1213, 196.8458) -> (171.0437, 196.9807) construction
  line L11563 (171.0437, 196.9807) -> (170.9678, 197.1168) construction
  line L11564 (170.9678, 197.1168) -> (170.8937, 197.2543) construction
  line L11565 (170.8937, 197.2543) -> (170.8214, 197.393) construction
  line L11566 (170.8214, 197.393) -> (170.7507, 197.5329) construction
  line L11567 (170.7507, 197.5329) -> (170.6816, 197.6738) construction
  line L11568 (170.6816, 197.6738) -> (170.6136, 197.8156) construction
  line L11569 (170.6136, 197.8156) -> (170.5467, 197.9581) construction
  line L11570 (170.5467, 197.9581) -> (170.4808, 198.1012) construction
  line L11571 (170.4808, 198.1012) -> (170.416, 198.245) construction
  line L11572 (170.416, 198.245) -> (170.3522, 198.3895) construction
  line L11573 (170.3522, 198.3895) -> (170.2896, 198.5347) construction
  line L11574 (170.2896, 198.5347) -> (170.2281, 198.6807) construction
  line L11575 (170.2281, 198.6807) -> (170.1678, 198.8274) construction
  line L11576 (170.1678, 198.8274) -> (170.1086, 198.9749) construction
  line L11577 (170.1086, 198.9749) -> (170.0505, 199.123) construction
  line L11578 (170.0505, 199.123) -> (169.9934, 199.2717) construction
  line L11579 (169.9934, 199.2717) -> (169.9373, 199.421) construction
  line L11580 (169.9373, 199.421) -> (169.8821, 199.5709) construction
  line L11581 (169.8821, 199.5709) -> (169.8279, 199.7214) construction
  line L11582 (169.8279, 199.7214) -> (169.7746, 199.8724) construction
  line L11583 (169.7746, 199.8724) -> (169.7223, 200.024) construction
  line L11584 (169.7223, 200.024) -> (169.671, 200.1761) construction
  line L11585 (169.671, 200.1761) -> (169.6206, 200.3288) construction
  line L11586 (169.6206, 200.3288) -> (169.5712, 200.482) construction
  line L11587 (169.5712, 200.482) -> (169.5226, 200.6358) construction
  line L11588 (169.5226, 200.6358) -> (169.475, 200.79) construction
  line L11589 (169.475, 200.79) -> (169.4283, 200.9447) construction
  line L11590 (169.4283, 200.9447) -> (169.3825, 201.0999) construction
  line L11591 (169.3825, 201.0999) -> (169.3375, 201.2556) construction
  line L11592 (169.3375, 201.2556) -> (169.2934, 201.4118) construction
  line L11593 (169.2934, 201.4118) -> (169.2502, 201.5684) construction
  line L11594 (169.2502, 201.5684) -> (169.2079, 201.7255) construction
  line L11595 (169.2079, 201.7255) -> (169.1664, 201.883) construction
  line L11596 (169.1664, 201.883) -> (169.1257, 202.0409) construction
  line L11597 (169.1257, 202.0409) -> (169.0859, 202.1993) construction
  line L11598 (169.0859, 202.1993) -> (169.047, 202.3581) construction
  line L11599 (169.047, 202.3581) -> (169.0089, 202.5173) construction
  line L11600 (169.0089, 202.5173) -> (168.9716, 202.6769) construction
  line L11601 (168.9716, 202.6769) -> (168.9351, 202.8369) construction
  line L11602 (168.9351, 202.8369) -> (168.8994, 202.9973) construction
  line L11603 (168.8994, 202.9973) -> (168.8646, 203.1581) construction
  line L11604 (168.8646, 203.1581) -> (168.8305, 203.3193) construction
  line L11605 (168.8305, 203.3193) -> (168.7973, 203.4809) construction
  line L11606 (168.7973, 203.4809) -> (168.7648, 203.6428) construction
  line L11607 (168.7648, 203.6428) -> (168.7332, 203.8051) construction
  line L11608 (168.7332, 203.8051) -> (168.7023, 203.9677) construction
  line L11609 (168.7023, 203.9677) -> (168.6723, 204.1307) construction
  line L11610 (168.6723, 204.1307) -> (168.643, 204.294) construction
  line L11611 (168.643, 204.294) -> (168.6145, 204.4577) construction
  line L11612 (168.6145, 204.4577) -> (168.5867, 204.6217) construction
  line L11613 (168.5867, 204.6217) -> (168.5597, 204.7861) construction
  line L11614 (168.5597, 204.7861) -> (168.5336, 204.9508) construction
  line L11615 (168.5336, 204.9508) -> (168.5081, 205.1158) construction
  line L11616 (168.5081, 205.1158) -> (168.4834, 205.2811) construction
  line L11617 (168.4834, 205.2811) -> (168.4595, 205.4467) construction
  line L11618 (168.4595, 205.4467) -> (168.4364, 205.6126) construction
  line L11619 (168.4364, 205.6126) -> (168.414, 205.7789) construction
  line L11620 (168.414, 205.7789) -> (168.3923, 205.9454) construction
  line L11621 (168.3923, 205.9454) -> (168.3714, 206.1122) construction
  line L11622 (168.3714, 206.1122) -> (168.3553, 206.2459) construction
  line L11623 (168.3553, 206.2459) -> (168.3435, 206.3463) construction
  line L11624 (168.3435, 206.3463) -> (168.3358, 206.4133) construction
  line L11625 (168.3358, 206.4133) -> (168.332, 206.4469) construction
  arc A309 (268.5789, 106.2) -> (271.2313, 109.8508) centre (212.132, 150) ccw
  spline S155 degree 5 poles (252.4583, 104.1847) (252.4787, 104.1615) (252.5188, 104.1146) (252.5771, 104.0427) (252.6512, 103.944) (252.7386, 103.8167) (252.8224, 103.6865) (252.904, 103.5546) (252.9844, 103.4218) (253.064, 103.2883) (253.1427, 103.1542) (253.2203, 103.0193) (253.2962, 102.8832) (253.3703, 102.7457) (253.4426, 102.607) (253.5133, 102.4671) (253.5824, 102.3262) (253.6504, 102.1844) (253.7173, 102.0419) (253.7832, 101.8988) (253.848, 101.755) (253.9118, 101.6105) (253.9744, 101.4653) (254.0359, 101.3193) (254.0962, 101.1726) (254.1554, 101.0251) (254.2135, 100.877) (254.2706, 100.7283) (254.3267, 100.579) (254.3819, 100.4291) (254.4361, 100.2786) (254.4894, 100.1276) (254.5417, 99.976) (254.593, 99.8239) (254.6434, 99.6712) (254.6928, 99.518) (254.7414, 99.3642) (254.789, 99.21) (254.8357, 99.0553) (254.8815, 98.9001) (254.9265, 98.7444) (254.9706, 98.5882) (255.0138, 98.4316) (255.0561, 98.2745) (255.0976, 98.117) (255.1383, 97.9591) (255.1781, 97.8007) (255.217, 97.6419) (255.2551, 97.4827) (255.2924, 97.3231) (255.3289, 97.1631) (255.3646, 97.0027) (255.3994, 96.8419) (255.4335, 96.6807) (255.4667, 96.5191) (255.4992, 96.3572) (255.5308, 96.1949) (255.5617, 96.0323) (255.5917, 95.8693) (255.621, 95.706) (255.6495, 95.5423) (255.6773, 95.3783) (255.7043, 95.2139) (255.7304, 95.0492) (255.7559, 94.8842) (255.7806, 94.7189) (255.8045, 94.5533) (255.8276, 94.3874) (255.85, 94.2211) (255.8717, 94.0546) (255.8926, 93.8878) (255.9087, 93.7541) (255.9205, 93.6537) (255.9282, 93.5867) (255.932, 93.5531) knots 0 0 0 0 0 0 0.01428571 0.02857143 0.04285714 0.05714286 0.07142857 0.08571429 0.1 0.11428571 0.12857143 0.14285714 0.15714286 0.17142857 0.18571429 0.2 0.21428571 0.22857143 0.24285714 0.25714286 0.27142857 0.28571429 0.3 0.31428571 0.32857143 0.34285714 0.35714286 0.37142857 0.38571429 0.4 0.41428571 0.42857143 0.44285714 0.45714286 0.47142857 0.48571429 0.5 0.51428571 0.52857143 0.54285714 0.55714286 0.57142857 0.58571429 0.6 0.61428571 0.62857143 0.64285714 0.65714286 0.67142857 0.68571429 0.7 0.71428571 0.72857143 0.74285714 0.75714286 0.77142857 0.78571429 0.8 0.81428571 0.82857143 0.84285714 0.85714286 0.87142857 0.88571429 0.9 0.91428571 0.92857143 0.94285714 0.95714286 0.97142857 0.98571429 1 1 1 1 1 1
  line L11626 (252.4583, 104.1847) -> (252.4787, 104.1615) construction
  line L11627 (252.4787, 104.1615) -> (252.5188, 104.1146) construction
  line L11628 (252.5188, 104.1146) -> (252.5771, 104.0427) construction
  line L11629 (252.5771, 104.0427) -> (252.6512, 103.944) construction
  line L11630 (252.6512, 103.944) -> (252.7386, 103.8167) construction
  line L11631 (252.7386, 103.8167) -> (252.8224, 103.6865) construction
  line L11632 (252.8224, 103.6865) -> (252.904, 103.5546) construction
  line L11633 (252.904, 103.5546) -> (252.9844, 103.4218) construction
  line L11634 (252.9844, 103.4218) -> (253.064, 103.2883) construction
  line L11635 (253.064, 103.2883) -> (253.1427, 103.1542) construction
  line L11636 (253.1427, 103.1542) -> (253.2203, 103.0193) construction
  line L11637 (253.2203, 103.0193) -> (253.2962, 102.8832) construction
  line L11638 (253.2962, 102.8832) -> (253.3703, 102.7457) construction
  line L11639 (253.3703, 102.7457) -> (253.4426, 102.607) construction
  line L11640 (253.4426, 102.607) -> (253.5133, 102.4671) construction
  line L11641 (253.5133, 102.4671) -> (253.5824, 102.3262) construction
  line L11642 (253.5824, 102.3262) -> (253.6504, 102.1844) construction
  line L11643 (253.6504, 102.1844) -> (253.7173, 102.0419) construction
  line L11644 (253.7173, 102.0419) -> (253.7832, 101.8988) construction
  line L11645 (253.7832, 101.8988) -> (253.848, 101.755) construction
  line L11646 (253.848, 101.755) -> (253.9118, 101.6105) construction
  line L11647 (253.9118, 101.6105) -> (253.9744, 101.4653) construction
  line L11648 (253.9744, 101.4653) -> (254.0359, 101.3193) construction
  line L11649 (254.0359, 101.3193) -> (254.0962, 101.1726) construction
  line L11650 (254.0962, 101.1726) -> (254.1554, 101.0251) construction
  line L11651 (254.1554, 101.0251) -> (254.2135, 100.877) construction
  line L11652 (254.2135, 100.877) -> (254.2706, 100.7283) construction
  line L11653 (254.2706, 100.7283) -> (254.3267, 100.579) construction
  line L11654 (254.3267, 100.579) -> (254.3819, 100.4291) construction
  line L11655 (254.3819, 100.4291) -> (254.4361, 100.2786) construction
  line L11656 (254.4361, 100.2786) -> (254.4894, 100.1276) construction
  line L11657 (254.4894, 100.1276) -> (254.5417, 99.976) construction
  line L11658 (254.5417, 99.976) -> (254.593, 99.8239) construction
  line L11659 (254.593, 99.8239) -> (254.6434, 99.6712) construction
  line L11660 (254.6434, 99.6712) -> (254.6928, 99.518) construction
  line L11661 (254.6928, 99.518) -> (254.7414, 99.3642) construction
  line L11662 (254.7414, 99.3642) -> (254.789, 99.21) construction
  line L11663 (254.789, 99.21) -> (254.8357, 99.0553) construction
  line L11664 (254.8357, 99.0553) -> (254.8815, 98.9001) construction
  line L11665 (254.8815, 98.9001) -> (254.9265, 98.7444) construction
  line L11666 (254.9265, 98.7444) -> (254.9706, 98.5882) construction
  line L11667 (254.9706, 98.5882) -> (255.0138, 98.4316) construction
  line L11668 (255.0138, 98.4316) -> (255.0561, 98.2745) construction
  line L11669 (255.0561, 98.2745) -> (255.0976, 98.117) construction
  line L11670 (255.0976, 98.117) -> (255.1383, 97.9591) construction
  line L11671 (255.1383, 97.9591) -> (255.1781, 97.8007) construction
  line L11672 (255.1781, 97.8007) -> (255.217, 97.6419) construction
  line L11673 (255.217, 97.6419) -> (255.2551, 97.4827) construction
  line L11674 (255.2551, 97.4827) -> (255.2924, 97.3231) construction
  line L11675 (255.2924, 97.3231) -> (255.3289, 97.1631) construction
  line L11676 (255.3289, 97.1631) -> (255.3646, 97.0027) construction
  line L11677 (255.3646, 97.0027) -> (255.3994, 96.8419) construction
  line L11678 (255.3994, 96.8419) -> (255.4335, 96.6807) construction
  line L11679 (255.4335, 96.6807) -> (255.4667, 96.5191) construction
  line L11680 (255.4667, 96.5191) -> (255.4992, 96.3572) construction
  line L11681 (255.4992, 96.3572) -> (255.5308, 96.1949) construction
  line L11682 (255.5308, 96.1949) -> (255.5617, 96.0323) construction
  line L11683 (255.5617, 96.0323) -> (255.5917, 95.8693) construction
  line L11684 (255.5917, 95.8693) -> (255.621, 95.706) construction
  line L11685 (255.621, 95.706) -> (255.6495, 95.5423) construction
  line L11686 (255.6495, 95.5423) -> (255.6773, 95.3783) construction
  line L11687 (255.6773, 95.3783) -> (255.7043, 95.2139) construction
  line L11688 (255.7043, 95.2139) -> (255.7304, 95.0492) construction
  line L11689 (255.7304, 95.0492) -> (255.7559, 94.8842) construction
  line L11690 (255.7559, 94.8842) -> (255.7806, 94.7189) construction
  line L11691 (255.7806, 94.7189) -> (255.8045, 94.5533) construction
  line L11692 (255.8045, 94.5533) -> (255.8276, 94.3874) construction
  line L11693 (255.8276, 94.3874) -> (255.85, 94.2211) construction
  line L11694 (255.85, 94.2211) -> (255.8717, 94.0546) construction
  line L11695 (255.8717, 94.0546) -> (255.8926, 93.8878) construction
  line L11696 (255.8926, 93.8878) -> (255.9087, 93.7541) construction
  line L11697 (255.9087, 93.7541) -> (255.9205, 93.6537) construction
  line L11698 (255.9205, 93.6537) -> (255.9282, 93.5867) construction
  line L11699 (255.9282, 93.5867) -> (255.932, 93.5531) construction
  spline S156 degree 5 poles (236.3268, 93.9655) (236.3391, 93.9372) (236.3628, 93.8802) (236.396, 93.7938) (236.4359, 93.6771) (236.4798, 93.5289) (236.5193, 93.3792) (236.5561, 93.2286) (236.5915, 93.0774) (236.626, 92.9259) (236.6594, 92.774) (236.6914, 92.6217) (236.7216, 92.4688) (236.7496, 92.3152) (236.7755, 92.1609) (236.7994, 92.006) (236.8217, 91.8506) (236.8425, 91.6948) (236.8621, 91.5386) (236.8805, 91.3821) (236.8978, 91.2253) (236.9138, 91.0682) (236.9285, 90.9107) (236.9418, 90.7529) (236.9538, 90.5947) (236.9645, 90.4362) (236.974, 90.2774) (236.9824, 90.1183) (236.9897, 89.9589) (236.9958, 89.7993) (237.0009, 89.6395) (237.0049, 89.4794) (237.0077, 89.3191) (237.0096, 89.1585) (237.0103, 88.9977) (237.01, 88.8367) (237.0086, 88.6755) (237.0062, 88.5141) (237.0028, 88.3525) (236.9985, 88.1907) (236.9931, 88.0288) (236.9868, 87.8666) (236.9795, 87.7043) (236.9712, 87.5419) (236.962, 87.3793) (236.9519, 87.2165) (236.9408, 87.0536) (236.9287, 86.8905) (236.9158, 86.7273) (236.902, 86.564) (236.8872, 86.4005) (236.8716, 86.2369) (236.855, 86.0732) (236.8376, 85.9094) (236.8193, 85.7455) (236.8001, 85.5815) (236.78, 85.4174) (236.7591, 85.2532) (236.7374, 85.0889) (236.7148, 84.9245) (236.6913, 84.76) (236.667, 84.5954) (236.6418, 84.4308) (236.6159, 84.266) (236.5891, 84.1013) (236.5614, 83.9364) (236.533, 83.7715) (236.5038, 83.6065) (236.4737, 83.4415) (236.4428, 83.2764) (236.4112, 83.1113) (236.3852, 82.9792) (236.3654, 82.8801) (236.352, 82.814) (236.3452, 82.7809) knots 0 0 0 0 0 0 0.01428571 0.02857143 0.04285714 0.05714286 0.07142857 0.08571429 0.1 0.11428571 0.12857143 0.14285714 0.15714286 0.17142857 0.18571429 0.2 0.21428571 0.22857143 0.24285714 0.25714286 0.27142857 0.28571429 0.3 0.31428571 0.32857143 0.34285714 0.35714286 0.37142857 0.38571429 0.4 0.41428571 0.42857143 0.44285714 0.45714286 0.47142857 0.48571429 0.5 0.51428571 0.52857143 0.54285714 0.55714286 0.57142857 0.58571429 0.6 0.61428571 0.62857143 0.64285714 0.65714286 0.67142857 0.68571429 0.7 0.71428571 0.72857143 0.74285714 0.75714286 0.77142857 0.78571429 0.8 0.81428571 0.82857143 0.84285714 0.85714286 0.87142857 0.88571429 0.9 0.91428571 0.92857143 0.94285714 0.95714286 0.97142857 0.98571429 1 1 1 1 1 1
  line L11700 (236.3268, 93.9655) -> (236.3391, 93.9372) construction
  line L11701 (236.3391, 93.9372) -> (236.3628, 93.8802) construction
  line L11702 (236.3628, 93.8802) -> (236.396, 93.7938) construction
  line L11703 (236.396, 93.7938) -> (236.4359, 93.6771) construction
  line L11704 (236.4359, 93.6771) -> (236.4798, 93.5289) construction
  line L11705 (236.4798, 93.5289) -> (236.5193, 93.3792) construction
  line L11706 (236.5193, 93.3792) -> (236.5561, 93.2286) construction
  line L11707 (236.5561, 93.2286) -> (236.5915, 93.0774) construction
  line L11708 (236.5915, 93.0774) -> (236.626, 92.9259) construction
  line L11709 (236.626, 92.9259) -> (236.6594, 92.774) construction
  line L11710 (236.6594, 92.774) -> (236.6914, 92.6217) construction
  line L11711 (236.6914, 92.6217) -> (236.7216, 92.4688) construction
  line L11712 (236.7216, 92.4688) -> (236.7496, 92.3152) construction
  line L11713 (236.7496, 92.3152) -> (236.7755, 92.1609) construction
  line L11714 (236.7755, 92.1609) -> (236.7994, 92.006) construction
  line L11715 (236.7994, 92.006) -> (236.8217, 91.8506) construction
  line L11716 (236.8217, 91.8506) -> (236.8425, 91.6948) construction
  line L11717 (236.8425, 91.6948) -> (236.8621, 91.5386) construction
  line L11718 (236.8621, 91.5386) -> (236.8805, 91.3821) construction
  line L11719 (236.8805, 91.3821) -> (236.8978, 91.2253) construction
  line L11720 (236.8978, 91.2253) -> (236.9138, 91.0682) construction
  line L11721 (236.9138, 91.0682) -> (236.9285, 90.9107) construction
  line L11722 (236.9285, 90.9107) -> (236.9418, 90.7529) construction
  line L11723 (236.9418, 90.7529) -> (236.9538, 90.5947) construction
  line L11724 (236.9538, 90.5947) -> (236.9645, 90.4362) construction
  line L11725 (236.9645, 90.4362) -> (236.974, 90.2774) construction
  line L11726 (236.974, 90.2774) -> (236.9824, 90.1183) construction
  line L11727 (236.9824, 90.1183) -> (236.9897, 89.9589) construction
  line L11728 (236.9897, 89.9589) -> (236.9958, 89.7993) construction
  line L11729 (236.9958, 89.7993) -> (237.0009, 89.6395) construction
  line L11730 (237.0009, 89.6395) -> (237.0049, 89.4794) construction
  line L11731 (237.0049, 89.4794) -> (237.0077, 89.3191) construction
  line L11732 (237.0077, 89.3191) -> (237.0096, 89.1585) construction
  line L11733 (237.0096, 89.1585) -> (237.0103, 88.9977) construction
  line L11734 (237.0103, 88.9977) -> (237.01, 88.8367) construction
  line L11735 (237.01, 88.8367) -> (237.0086, 88.6755) construction
  line L11736 (237.0086, 88.6755) -> (237.0062, 88.5141) construction
  line L11737 (237.0062, 88.5141) -> (237.0028, 88.3525) construction
  line L11738 (237.0028, 88.3525) -> (236.9985, 88.1907) construction
  line L11739 (236.9985, 88.1907) -> (236.9931, 88.0288) construction
  line L11740 (236.9931, 88.0288) -> (236.9868, 87.8666) construction
  line L11741 (236.9868, 87.8666) -> (236.9795, 87.7043) construction
  line L11742 (236.9795, 87.7043) -> (236.9712, 87.5419) construction
  line L11743 (236.9712, 87.5419) -> (236.962, 87.3793) construction
  line L11744 (236.962, 87.3793) -> (236.9519, 87.2165) construction
  line L11745 (236.9519, 87.2165) -> (236.9408, 87.0536) construction
  line L11746 (236.9408, 87.0536) -> (236.9287, 86.8905) construction
  line L11747 (236.9287, 86.8905) -> (236.9158, 86.7273) construction
  line L11748 (236.9158, 86.7273) -> (236.902, 86.564) construction
  line L11749 (236.902, 86.564) -> (236.8872, 86.4005) construction
  line L11750 (236.8872, 86.4005) -> (236.8716, 86.2369) construction
  line L11751 (236.8716, 86.2369) -> (236.855, 86.0732) construction
  line L11752 (236.855, 86.0732) -> (236.8376, 85.9094) construction
  line L11753 (236.8376, 85.9094) -> (236.8193, 85.7455) construction
  line L11754 (236.8193, 85.7455) -> (236.8001, 85.5815) construction
  line L11755 (236.8001, 85.5815) -> (236.78, 85.4174) construction
  line L11756 (236.78, 85.4174) -> (236.7591, 85.2532) construction